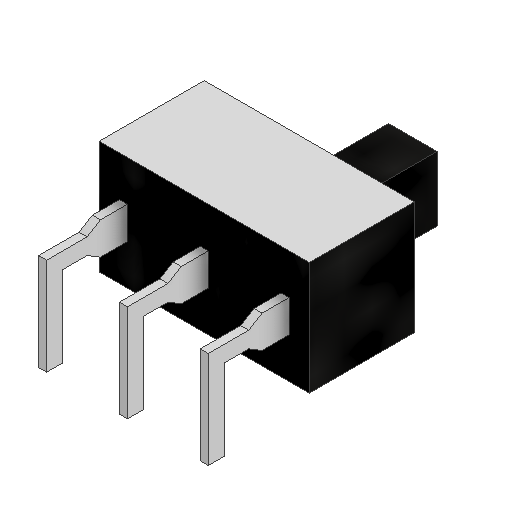
# Autodesk Inventor part: Switch
Saved by Autodesk Inventor 2025.2 (Build 292293000, 293)
## iProperties
Created: 2025-03-09
Part Number: Switch
Material: Generic
Document SubType Name: Modeling
Designer: ahorat
Density: 1 g/cm^3
Appearance: Default
Author: ahorat
Autodesk Inventor part; units mm, degrees
ref_plane "YZ Plane" through (0, 0, 0) normal (1, 0, 0) x (0, 1, 0)
ref_plane "XZ Plane" through (0, 0, 0) normal (0, 1, 0) x (-1, 0, 0)
ref_plane "XY Plane" through (0, 0, 0) normal (0, 0, 1) x (1, 0, 0)
sketch "Sketch1" plane through (0, 0, 0) normal (0, 0, 1) x (1, 0, 0)
  line L0 (-6.5, 0) -> (6.5, 0)
  line L1 (6.5, 0) -> (6.5, 7)
  line L2 (6.5, 7) -> (-6.5, 7)
  line L3 (-6.5, 7) -> (-6.5, 0)
  point P0 (0, 0)
  point P1 (0, 0)
  dimension "d0" = 13
  dimension "d1" = 7
  constraints: 8 end point, 2 parallel, 1 coincident, 1 horizontal, 1 midpoint, 1 perpendicular
  measures "d0" distance of L1.end L2.end
  measures "d1" distance of L0.end L1.end
extrude "Extrusion1" add sketch "Sketch1" along normal blind 6.5
sketch "Sketch2" plane through (0, 0, 0) normal (0, 0, -1) x (-1, 0, 0)
  line L0 (-3, 5.5) -> (3, 5.5)
  line L1 (3, 5.5) -> (3, 1.5)
  line L2 (3, 1.5) -> (-3, 1.5)
  line L3 (-3, 1.5) -> (-3, 5.5)
  line L4 (6.5, 0) -> (-6.5, 0) projected
  line L5 (-6.5, 0) -> (-6.5, 7) projected
  point P0 (0, 0)
  point P1 (0, 1.5)
  point P2 (0, 0)
  point P3 (-3, 3.5)
  point P4 (-6.5, 3.5)
  dimension "d4" = 4
  dimension "d5" = 6
  constraints: 8 end point, 4 midpoint, 2 parallel, 1 horizontal, 1 horizontal alignment, 1 perpendicular, 1 vertical alignment
  measures "d4" distance of L0.end L1.end
  measures "d5" distance of L0.start L0.end
extrude "Extrusion2" cut sketch "Sketch2" against normal blind 0.1
sketch "Sketch3" plane through (0, 0, 0.1) normal (0, 0, -1) x (-1, 0, 0)
  line L0 (-3, 1.5) -> (-3, 5.5) projected
  line L1 (3, 1.5) -> (-3, 1.5) projected
  line L2 (-3, 5.5) -> (0, 5.5)
  line L3 (0, 5.5) -> (0, 1.5)
  line L4 (0, 1.5) -> (-3, 1.5)
  line L5 (-3, 1.5) -> (-3, 5.5)
  point P0 (0, 0)
  constraints: 8 end point, 2 parallel, 1 horizontal, 1 midpoint, 1 perpendicular
extrude "Extrusion3" add sketch "Sketch3" along normal blind 5
sketch "Sketch4" plane through (0, 0, 0) normal (1, 0, 0) x (0, 1, 0)
  line L0 (0, 6.5) -> (7, 6.5) projected
  line L1 (4, 6.5) -> (4, 11.5)
  line L2 (4, 11.5) -> (-2, 11.5)
  line L3 (-2, 11.5) -> (-2, 10.5)
  line L4 (-2, 10.5) -> (3, 10.5)
  line L5 (3, 10.5) -> (3, 6.5)
  line L6 (3, 9) -> (2.5, 8.1738)
  line L7 (2.5, 8.1738) -> (2.5, 6.5)
  line L8 (4, 9) -> (4.5, 8.1738)
  line L9 (4.5, 8.1738) -> (4.5, 6.5)
  line L10 (0, 0) -> (0, 6.5) projected
  line L11 (4, 9) -> (3, 9) construction
  point P0 (-2, 11)
  point P1 (3.5, 9)
  point P2 (3.5, 6.5)
  dimension "d10" = 1
  dimension "d11" = 1
  dimension "d12" = 2
  dimension "d13" = 2
  dimension "d14" = 5
  constraints: 20 end point, 5 point on line, 4 midpoint, 4 perpendicular, 2 horizontal alignment, 2 parallel, 1 equal length, 1 horizontal, 1 vertical, 1 vertical alignment
  measures "d10" distance between parallel lines of L1 L5
  measures "d11" distance between parallel lines of L4 L2
  measures "d12" distance between parallel lines of L9 L7
  measures "d13" distance from line of point (-2, 11) L10
  measures "d14" distance between parallel lines of L0 L2
extrude "Extrusion4" add sketch "Sketch4" along normal mid plane 0.5
pattern_linear "Rectangular Pattern1" count 2 spacing 5 along (-1, 0, 0) of "Extrusion4"
mirror "Mirror1" about plane through (0, 0, 0) normal (1, 0, 0) of "Extrusion4", "Rectangular Pattern1"
body "Solid1"
